marlin ramps lcd (Autodesk Fusion 360 design; units mm, degrees)
Autodesk Fusion 360 part; units mm, degrees
sketch "Sketch1" plane through (0, 0, 0) normal (0, 1, 0) x (1, 0, 0)
  line L0 (98, 0) -> (98, -44)
  line L1 (98, -44) -> (98, -42)
  line L2 (124, -19) -> (124, -37)
  line L3 (0, -42) -> (98, -42)
  line L4 (2, -44) -> (2, 0)
  circle A0 centre (124, -18) radius 5
  line L5 (124, -18) -> (124, -35)
  circle A1 centre (124, -35) radius 4
  line L6 (2, 0) -> (2, -2)
  line L7 (2, -2) -> (98, -2)
  line L8 (2, -2) -> (2, -42)
  dimension "d3" = 2
  dimension "d4" = 96
  dimension "d6" = 2
  dimension "d16" = 10
  dimension "d17" = 17
  dimension "d18" = 8
  constraint coincident A0.centre L5.start
  constraint coincident L5.end A1.centre
  constraint coincident L0 L7.end
  constraint perpendicular L0 L7
  constraint coincident L3 L8.end
  constraint coincident L4 L8.end
  constraint perpendicular L3 L8
  measures "d3" distance of origin L4.end
  measures "d4" distance of L4.end L0.start
  measures "d6" distance of L0.end L1.end
  measures "d16" diameter of A0
  measures "d17" distance of A0.centre L5.end
  measures "d18" diameter of A1
extrude "Extrude1" add sketch "Sketch1" along normal blind 40 makes body 1 at (34, 13.3333, 42) makes body 2 at (128.9752, 26.6667, 17.5022) makes body 3 at (127.9801, 26.6667, 34.6017)
sketch "Sketch2" plane through (0, 40, 0) normal (0, 1, 0) x (-1, 0, 0)
  line L0 (-99, 43) -> (-1, 43)
  line L1 (-1, 43) -> (-1, 1)
  line L2 (-1, 1) -> (-99, 1)
  line L3 (-99, 1) -> (-99, 43)
extrude "Extrude2" add sketch "Sketch2" against normal blind 40 separate body makes body 4
copy_body "CutPasteBodies1" bodies 2 removing the originals makes body 5 in component "main hole"
copy_body "CutPasteBodies2" bodies 3 removing the originals makes body 6 in component "main hole"
copy_body "CutPasteBodies3" bodies 4 removing the originals makes body 7 in component "main hole"
sketch "Sketch1 (2)" plane through (0, 40, 0) normal (0, 1, 0) x (-1, 0, 0) in component "shell"
  line L0 (-99, 1) -> (-1, 1)
  line L1 (-1, 1) -> (-1, 43)
  line L2 (-1, 43) -> (-99, 43)
  line L3 (-99, 43) -> (-99, 1)
  line L4 (-1, 43) -> (13, 43)
  line L5 (-99, 43) -> (-99, 54)
  line L6 (-99, 1) -> (-99, -11)
  line L7 (-99, 1) -> (-138, 1)
  line L8 (-138, -11) -> (13, -11)
  line L9 (13, -11) -> (13, 54)
  line L10 (13, 54) -> (-138, 54)
  line L11 (-138, 54) -> (-138, -11)
  line L12 (-139, -12) -> (14, -12)
  line L13 (14, -12) -> (14, 55)
  line L14 (14, 55) -> (-139, 55)
  line L15 (-139, 55) -> (-139, -12)
  line L16 (-140, -13) -> (15, -13)
  line L17 (15, -13) -> (15, 56)
  line L18 (15, 56) -> (-140, 56)
  line L19 (-140, 56) -> (-140, -13)
  dimension "d29" = 14
  dimension "d30" = 11
  dimension "d31" = 12
  dimension "d32" = 39
  dimension "d33" = 1
  dimension "d34" = 2
  constraint coincident L1.end L2.start
  constraint perpendicular L1 L4
  constraint coincident L2.end L3.start
  constraint perpendicular L2 L5
  constraint coincident L0.start L3.end
  constraint perpendicular L0 L6
  constraint perpendicular L6 L7
  constraint horizontal L8
  constraint vertical L9
  constraint horizontal L10
  constraint vertical L11
  measures "d29" distance of L1.end L4.end
  measures "d30" distance of L2.end L5.end
  measures "d31" distance of L0.start L6.end
  measures "d32" distance of L0.start L7.end
extrude "Extrude1'" add sketch "Sketch1 (2)" against normal blind 40 separate body contours L16 L17 L18 L19 makes body 8 in component "shell"
sketch "Sketch5" plane through (0, 40, 0) normal (0, 1, 0) x (-1, 0, 0) in component "shell"
  line L0 (15, -13) -> (-140, -13)
  line L1 (-140, -13) -> (-140, 56)
  line L2 (-140, 56) -> (15, 56)
  line L3 (15, 56) -> (15, -13)
  constraint horizontal L0
  constraint vertical L1
  constraint horizontal L2
  constraint vertical L3
extrude "Extrude1''" add sketch "Sketch5" against normal blind 1 separate body makes body 9 in component "face"
combine "Combine1" operation cut target body 9 tool bodies 6 7 5 in component "face"
combine "Combine1'" operation add target body 9 tool bodies 8 keep tools result as body 10 in component "Component"
sketch "Sketch1 (3)" plane through (0, 39, 0) normal (0, -1, 0) x (1, 0, 0) in component "Component"
  line L0 (139, 55) -> (-14, 55)
  line L1 (-14, 55) -> (-14, -12)
  line L2 (-14, -12) -> (139, -12)
  line L3 (139, -12) -> (139, 55)
  circle A0 centre (124, 18) radius 5
  line L4 (1, 1) -> (1, 43)
  line L5 (1, 43) -> (99, 43)
  line L6 (99, 43) -> (99, 1)
  line L7 (99, 1) -> (1, 1)
  circle A1 centre (124, 35) radius 4
  line L8 (99, 22) -> (104, 22)
  line L9 (1, 22) -> (-4, 22)
  line L10 (104, 22) -> (104, 43)
  line L11 (104, 43) -> (104, 1)
  line L12 (104, 43) -> (109, 43)
  line L13 (109, 43) -> (109, 1)
  line L14 (109, 1) -> (104, 1)
  line L15 (104, 1) -> (104, 43)
  line L16 (-4, 22) -> (-4, 43)
  line L17 (-4, 43) -> (-4, 1)
  line L18 (-4, 1) -> (-9, 1)
  line L19 (-9, 1) -> (-9, 43)
  line L20 (-9, 43) -> (-4, 43)
  line L21 (-4, 43) -> (-4, 1)
  dimension "d39" = 5
  dimension "d40" = 5
  dimension "d41" = 42
  dimension "d42" = 5
  dimension "d43" = 5
  constraint midpoint L6 L8.start
  constraint perpendicular L3 L8
  constraint midpoint L4 L9.start
  constraint perpendicular L4 L9
  constraint perpendicular L5 L10
  constraint perpendicular L5 L11
  constraint horizontal L12
  constraint vertical L13
  constraint horizontal L14
  constraint vertical L15
  constraint perpendicular L5 L16
  constraint perpendicular L5 L17
  constraint horizontal L18
  constraint vertical L19
  constraint horizontal L20
  constraint vertical L21
  measures "d39" distance of L8.start L8.end
  measures "d40" distance of L9.start L9.end
  measures "d41" distance of L10.end L11.end
  measures "d42" distance of L10.end L12.end
  measures "d43" distance of L17.end L18.end
extrude "Extrude1'''" add sketch "Sketch1 (3)" along normal blind 10 contours L10 L11 L12 L13 L14 L15 | L16 L17 L18 L19 L20 L21 bodies 10 in component "Component"
chamfer "Chamfer1" distance 5 angle 45 4 edges at (62.5, 39, -12) (139, 39, 21.5) (62.5, 39, 55) (-14, 39, 21.5) on bodies 10 in component "Component"
sketch "Sketch2 (2)" plane through (-15, 0, 0) normal (-1, 0, 0) x (0, 0, 1) in component "Component"
  line L0 (56, 40) -> (-13, 40)
  line L1 (-13, 40) -> (-13, 0)
  line L2 (-13, 0) -> (56, 0)
  line L3 (56, 0) -> (56, 40)
  line L4 (-13, 40) -> (-13, 25)
  line L5 (-13, 25) -> (56, 25)
  line L6 (1, -1) -> (-13, 0)
  line L7 (1.0019, 40) -> (-13, 40)
  line L8 (42.9868, 40) -> (56, 40)
  line L9 (42.9868, 40) -> (42.9868, 25)
  line L10 (1.0019, 40) -> (1.0019, 25)
  line L11 (1.0019, 25) -> (42.9868, 25)
  line L12 (42.9868, 25) -> (42.9868, 20)
  line L13 (42.9868, 20) -> (1.0019, 20)
  line L14 (1.0019, 20) -> (1.0019, 25)
  line L15 (1.0019, 20) -> (4.0019, 20)
  line L16 (42.9868, 20) -> (39.9868, 20)
  line L17 (4.0019, 20) -> (40, 20)
  line L18 (40, 20) -> (40, 25)
  line L19 (40, 25) -> (4.0019, 25)
  line L20 (4.0019, 25) -> (4.0019, 20)
  dimension "d47" = 15
  dimension "d48" = 5
  dimension "d49" = 3
  dimension "d50" = 3
  constraint coincident L0.end L1.start
  constraint perpendicular L0 L4
  constraint horizontal L5
  constraint coincident L3 L5.end
  constraint coincident L1.end L2.start
  constraint coincident L0 L7.start
  constraint perpendicular L4 L7
  constraint coincident L0 L8.start
  constraint coincident L0.start L3.end
  constraint parallel L0 L8
  constraint coincident L5 L9.end
  constraint perpendicular L5 L9
  constraint coincident L5 L10.end
  constraint perpendicular L5 L10
  constraint horizontal L11
  constraint vertical L12
  constraint horizontal L13
  constraint vertical L14
  constraint perpendicular L14 L15
  constraint perpendicular L12 L16
  constraint horizontal L17
  constraint vertical L18
  constraint horizontal L19
  constraint vertical L20
  constraint coincident L5 L18.end
  measures "d47" distance of L0.end L4.end
  measures "d48" distance of L10.end L13.end
  measures "d49" distance of L13.end L15.end
  measures "d50" distance of L12.end L16.end
extrude "Extrude2'" cut sketch "Sketch2 (2)" against normal blind 10 contours L5 L11 L13 L16 L17 L18 L19 L20 bodies 10 in component "Component"
extrude "Extrude3" cut 1 faces at (88, 0, 55.6667) along direction (0, 1, 0) blind 15 on bodies 10 bodies 10 in component "Component"
component "main hole" placed x (1, 0, 0) y (0, 1, 0) z (0, 0, 1) at (0, 0, 0)
component "shell" placed x (1, 0, 0) y (0, 1, 0) z (0, 0, 1) at (0, 0, 0)
component "Component" placed x (1, 0, 0) y (0, 1, 0) z (0, 0, 1) at (5.1837, 6.851, -5.8681)
component "face" placed x (1, 0, 0) y (0, 1, 0) z (0, 0, 1) at (0, 0, 0) in component "shell"
hidden bodies 1
named bodies: "lcd"
